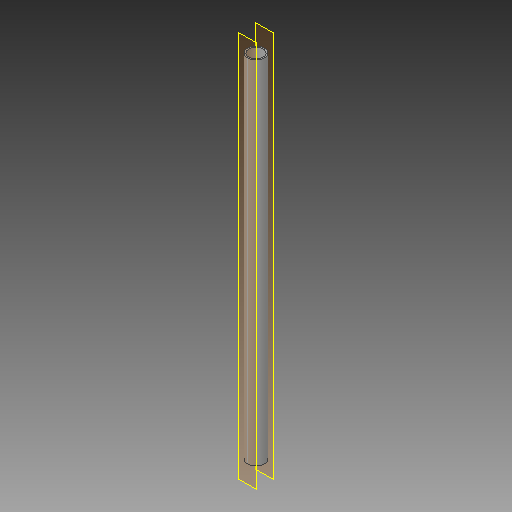
# Autodesk Inventor part: rør
Saved by Autodesk Inventor 2018 (Build 220112000, 112)
## iProperties
Created: 2019-09-25
Part Number: rør
Material: Steel
Document SubType Name: Modeling
Designer: loppen
Density: 7.85 g/cm^3
Appearance: Light Gray
Mass: 4138.51 g
Surface Area: 2822.27 cm^2
Volume: 527.199 cm^3
Author: loppen
Autodesk Inventor part; units mm, degrees
ref_plane "YZ Plane" through (0, 0, 0) normal (1, 0, 0) x (0, 1, 0)
ref_plane "XZ Plane" through (0, 0, 0) normal (0, 1, 0) x (-1, 0, 0)
sketch "Sketch1" plane through (0, 0, 0) normal (0, 1, 0) x (-1, 0, 0)
  circle A0 centre (0, 0) radius 24.25
  circle A1 centre (0, 0) radius 20.5
  dimension "d0" = 48.5
  dimension "d1" = 3.75
  dimension "d2" = 41
  constraints: 2 centre point, 2 coincident
  measures "d0" diameter of A0
  measures "d1" radial gap between concentric circles of A0 A1
  measures "d2" diameter of A1
extrude "Extrusion1" add sketch "Sketch1" along normal blind 1000
ref_plane "rørtangent 1" through (0, 0, 24.25) normal (0, 0, 1) x (1, 0, 0)
ref_plane "rørtangent 2" through (0, 0, -24.25) normal (0, 0, 1) x (1, 0, 0)
body "Solid1"
